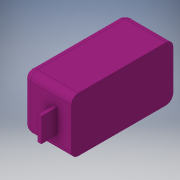
# Autodesk Inventor part: LIDAR-LITE V4
Saved by Autodesk Inventor 2019 (Build 230136000, 136)
## iProperties
Created: 2020-08-15
Part Number: LIDAR-LITE V4
Material: Generic
Document SubType Name: Modeling
Designer: james
Density: 1 g/cm^3
Appearance: Default(1)
Author: james
Autodesk Inventor part; units mm, degrees
ref_plane "YZ Plane" through (0, 0, 0) normal (1, 0, 0) x (0, 1, 0)
ref_plane "XZ Plane" through (0, 0, 0) normal (0, 1, 0) x (-1, 0, 0)
ref_plane "XY Plane" through (0, 0, 0) normal (0, 0, 1) x (1, 0, 0)
sketch "Sketch1" plane through (0, 0, 0) normal (1, 0, 0) x (0, 1, 0)
  line L0 (13.8453, 20.5662) -> (-10.1847, 20.5662)
  line L1 (-10.1847, 20.5662) -> (-10.1847, -24.4138)
  line L2 (-10.1847, -24.4138) -> (13.8453, -24.4138)
  line L3 (13.8453, -24.4138) -> (13.8453, 20.5662)
  point P0 (0, 0)
  dimension "d0" = 24.03
  dimension "d1" = 44.98
  constraints: 8 end point, 2 parallel, 1 horizontal, 1 perpendicular
  measures "d0" distance of L1.end L2.end
  measures "d1" distance of L0.end L1.end
extrude "Extrusion1" add sketch "Sketch1" along normal blind 15.2
fillet "Fillet1" radius 3.175 8 edges at (7.6, 13.8453, 20.5662) (7.6, -10.1847, 20.5662) (7.6, 13.8453, -24.4138) (7.6, -10.1847, -24.4138) (0, 1.8303, -24.4138) (0, 13.8453, -1.9238) (0, -10.1847, -1.9238) (0, 1.8303, 20.5662)
sketch "Sketch2" plane through (15.2, 0, 0) normal (1, 0, 0) x (0, 0, -1)
  line L0 (-20.5662, -7.0097) -> (-20.5662, 10.6703) projected
  line L1 (-27.7562, 7.1303) -> (-20.5662, 7.1303)
  line L2 (-20.5662, 7.1303) -> (-20.5662, -3.4697)
  line L3 (-20.5662, -3.4697) -> (-27.7562, -3.4697)
  line L4 (-27.7562, -3.4697) -> (-27.7562, 7.1303)
  line L5 (21.2388, 13.8453) -> (-17.3912, 13.8453) projected
  point P0 (0, 0)
  dimension "d5" = 10.6
  dimension "d6" = 6.715
  dimension "d7" = 7.19
  constraints: 8 end point, 2 parallel, 1 horizontal, 1 perpendicular, 1 point on line
  measures "d5" distance of L3.end L1.start
  measures "d6" distance between parallel lines of L1 L5
  measures "d7" distance of L2.end L3.end
extrude "Extrusion2" add sketch "Sketch2" against normal blind 1.5
sketch "Sketch3" plane through (15.2, 0, 0) normal (1, 0, 0) x (0, 0, -1)
  line L0 (-17.3912, 10.6703) -> (-17.3912, -7.0097) projected
  line L1 (-20.5662, -3.4697) -> (-20.5662, -7.0097) projected
  line L2 (-20.5662, 10.6703) -> (-20.5662, 7.1303) projected
  arc A0 (-17.3912, 13.8453) -> (-20.5662, 10.6703) centre (-17.3912, 10.6703) ccw projected
  line L3 (21.2388, 13.8453) -> (-17.3912, 13.8453) projected
  line L4 (24.4138, -7.0097) -> (24.4138, 10.6703) projected
  arc A1 (24.4138, 10.6703) -> (21.2388, 13.8453) centre (21.2388, 10.6703) ccw projected
  arc A2 (21.2388, -10.1847) -> (24.4138, -7.0097) centre (21.2388, -7.0097) ccw projected
  line L5 (-17.3912, -10.1847) -> (21.2388, -10.1847) projected
  arc A3 (-20.5662, -7.0097) -> (-17.3912, -10.1847) centre (-17.3912, -7.0097) ccw projected
  line L6 (-20.5662, -10.1847) -> (21.2388, -10.1847)
  line L7 (24.4138, -7.0097) -> (24.4138, 13.8453)
  line L8 (24.4138, 13.8453) -> (-20.5662, 13.8453)
  line L9 (-20.5662, 13.8453) -> (-20.5662, -10.1847)
  line L10 (-17.3912, -7.0097) -> (21.2388, -7.0097) projected
  line L11 (21.2388, -7.0097) -> (21.2388, 10.6703) projected
  arc A4 (21.2388, -10.1847) -> (24.4138, -7.0097) centre (21.2388, -7.0097) ccw
  point P0 (0, 0)
  dimension "d10" = 0
  dimension "d11" = 0
  dimension "d12" = 0
  dimension "d13" = 0
  constraints: 9 end point, 4 point on circle, 2 parallel, 1 centre point, 1 coincident, 1 horizontal, 1 perpendicular
  measures "d10" distance between parallel lines of L9 L1
  measures "d11" distance between parallel lines of L6 L5
  measures "d12" distance between parallel lines of L4 L7
  measures "d13" distance between parallel lines of L3 L8
extrude "Extrusion3" add sketch "Sketch3" along normal blind 6
fillet "Fillet2" radius 3.175 3 edges at (18.2, -10.1847, 20.5662) (18.2, 13.8453, 20.5662) (18.2, 13.8453, -24.4138)
body "Solid1"
